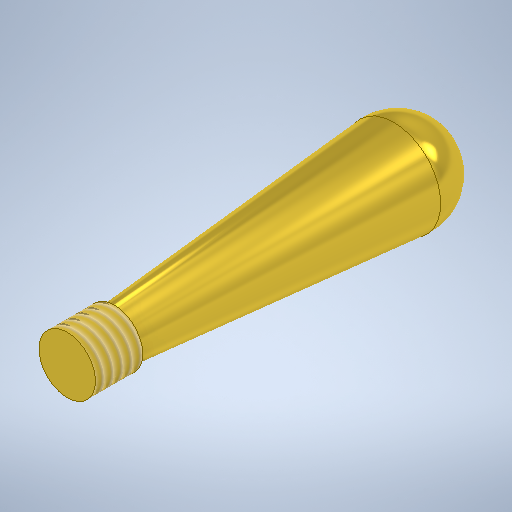
# Autodesk Inventor part: 134 handle
Saved by Autodesk Inventor 2025.1 (Build 291241000, 241)
## iProperties
Created: 2024-08-05
Part Number: 134 handle
Material: Lead
Document SubType Name: Modeling
Designer: ffogue
Density: 11.34 g/cm^3
Appearance: Metal 2400F Hot
Author: ffogue
Autodesk Inventor part; units mm, degrees
ref_plane "YZ Plane" through (0, 0, 0) normal (1, 0, 0) x (0, 1, 0)
ref_plane "XZ Plane" through (0, 0, 0) normal (0, 1, 0) x (-1, 0, 0)
ref_plane "XY Plane" through (0, 0, 0) normal (0, 0, 1) x (1, 0, 0)
sketch "Sketch1" plane through (0, 0, 0) normal (0, 0, 1) x (1, 0, 0)
  line L0 (0, 0) -> (0, 20)
  line L1 (0, 0) -> (1.5, 0)
  line L2 (1.5, 0) -> (1.5, 2.5)
  line L3 (1.5, 2.5) -> (1.25, 2.5)
  line L4 (1.25, 2.5) -> (2.4912, 17.2909)
  arc A0 (2.4912, 17.2909) -> (0, 20) centre (0, 17.5) ccw
  point P0 (0.75, 0)
  dimension "d0" = 3
  dimension "d3" = 2.5
  dimension "d5" = 20
  dimension "d6" = 2.5
  dimension "d9" = 2.5
  constraints: 10 end point, 2 perpendicular, 2 point on circle, 2 vertical alignment, 1 centre point, 1 horizontal, 1 midpoint, 1 tangent, 1 vertical
  measures "d0" diameter of L2 L0
  measures "d3" distance of L1.end L2.end
  measures "d5" distance from line of L1 L0.end
  measures "d6" radius of A0
  measures "d9" vertical distance of L3.end L0
revolve "Revolution1" add sketch "Sketch1" angle 360 about axis through (0, 0, 0) along (0, 1, 0)
thread "Thread1" size "M3x0.5" class "6g" standard "ISO Metric profile" length 10
body "Solid1"
